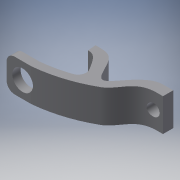
# Autodesk Inventor part: 30_Cube_Chipadapter_Fluicis_clamp
Saved by Autodesk Inventor 2019.4 (Build 234330000, 330)
## iProperties
Created: 2021-05-02
Part Number: 30_Cube_Chipadapter_Fluicis_clamp
Material: Generic
Document SubType Name: Modeling
Designer: diederichbenedict
Density: 1 g/cm^3
Appearance: Default
Author: diederichbenedict
Autodesk Inventor part; units mm, degrees
ref_plane "YZ Plane" through (0, 0, 0) normal (1, 0, 0) x (0, 1, 0)
ref_plane "XZ Plane" through (0, 0, 0) normal (0, 1, 0) x (-1, 0, 0)
ref_plane "XY Plane" through (0, 0, 0) normal (0, 0, 1) x (1, 0, 0)
sketch "Sketch1" plane through (0, 0, 0) normal (0, 1, 0) x (-1, 0, 0)
  line L0 (0, 0) -> (3.0089, 0) construction
  line L1 (3.0089, 0) -> (7.069, 5.8831) construction
  line L2 (7.069, 5.8831) -> (8.9606, 9.5326) construction
  line L3 (8.9606, 9.5326) -> (11.3861, 1.7338) construction
  line L4 (11.3861, 1.7338) -> (15.5604, 1.7338) construction
  spline S0 degree 4 poles (0, 0) (3.0089, 0) (7.069, 5.8831) (8.9606, 9.5326) (11.3861, 1.7338) (11.3861, 1.7338) (15.5604, 1.7338) knots 1 1 1 1 1 2 3 4 4 4 4 4
  line L5 (0, 0) -> (-2.509, 0)
  line L6 (-2.509, 0) -> (-2.509, 2.5)
  line L7 (-2.509, 2.5) -> (-1.0509, 2.5)
  line L8 (-1.0509, 2.5) -> (3.5176, 2.5) construction
  line L9 (3.5176, 2.5) -> (4.4785, 7.5024) construction
  line L10 (4.4785, 7.5024) -> (10.7757, 12.1884) construction
  line L11 (10.7757, 12.1884) -> (13.1491, 3.4753) construction
  line L12 (13.1491, 3.4753) -> (13.5495, 3.0077) construction
  line L13 (13.5495, 3.0077) -> (15.5604, 3.0077) construction
  spline S1 degree 4 poles (-1.0509, 2.5) (3.5176, 2.5) (4.4785, 7.5024) (10.7757, 12.1884) (13.1491, 3.4753) (13.5495, 3.0077) (15.5604, 3.0077) knots 1 1 1 1 1 2 3 4 4 4 4 4
  line L14 (15.5604, 3.0077) -> (15.5604, 1.7338)
  dimension "d0" = 2.5
  constraints: 8 end point, 5 horizontal, 2 perpendicular, 1 coincident, 6 other
  measures "d0" distance of L5.end L6.end
extrude "Extrusion1" add sketch "Sketch1" along normal blind 8
sketch "Sketch2" plane through (1.0509, 0, 2.5) normal (0, 0, 1) x (1, 0, 0)
  circle A0 centre (-0.8088, 4) radius 1.45
  line L0 (-16.6113, 8) -> (0, 8) projected
  point P0 (-1.0509, 0)
  dimension "d3" = 2.9
  dimension "d14" = 4
  constraints: 1 centre point
  measures "d3" diameter of A0
  measures "d14" distance from line of A0.centre L0
extrude "Extrusion2" cut sketch "Sketch2" along normal mid plane 7
sketch "Sketch3" plane through (0, 0, 0) normal (0, -1, 0) x (1, 0, 0)
  line L0 (2.509, 0) -> (0, 0) projected
  line L1 (2.509, 2.5) -> (2.509, 0) projected
  line L2 (1.0509, 2.5) -> (2.509, 2.5) projected
  spline S0 degree 4 poles (-15.5604, 3.0077) (-13.5495, 3.0077) (-13.1491, 3.4753) (-10.7757, 12.1884) (-4.4785, 7.5024) (-3.5176, 2.5) (1.0509, 2.5) knots 0 0 0 0 0 0.333333 0.666667 1 1 1 1 1 projected
  line L3 (-15.5604, 1.7338) -> (-15.5604, 3.0077) projected
  arc A0 (-7.1833, 8.351) -> (-19.9296, 12.3019) centre (-22.9296, -19.9129) ccw
  arc A1 (-10.767, 7.9081) -> (-19.9296, 10.3019) centre (-22.9296, -19.9129) ccw
  line L4 (-19.9296, 12.3019) -> (-19.9296, 10.3019)
  line L5 (-19.9296, 12.3019) -> (-25.9296, 12.3019)
  line L6 (-25.9296, 12.3019) -> (-25.9296, 10.3019)
  line L7 (-25.9296, 10.3019) -> (-19.9296, 10.3019)
  line L8 (-19.9296, 10.3019) -> (-19.9296, 12.3019)
  dimension "d6" = 6
  dimension "d7" = 2
  constraints: 10 end point, 5 point on circle, 2 centre point, 2 parallel, 1 concentric, 1 horizontal, 1 perpendicular, 5 other
  measures "d6" distance of L4.end L6.end
  measures "d7" distance between parallel lines of L7 L5
extrude "Extrusion3" add sketch "Sketch3" against normal up to surface (8 mm away)
sketch "Sketch4" plane through (-25.9296, 0, 12.3019) normal (0, 0, 1) x (1, 0, 0)
  arc A0 (0.3271, 6.628) -> (0.3271, 0.742) centre (3.8271, 3.685) ccw projected
  arc A1 (26.9804, 2.7965) -> (26.9804, 5.2035) centre (26.1717, 4) ccw projected
  circle A2 centre (3.8592, 4) radius 2.5
  point P0 (25.9296, 0)
  dimension "d10" = 5
  constraints: 1 centre point, 1 vertical alignment
  measures "d10" diameter of A2
extrude "Extrusion4" cut sketch "Sketch4" against normal blind 10
fillet "Fillet1" radius 2 3 edges at (-25.9296, 0, 11.3019) (-25.9296, 8, 11.3019) (-10.767, 4, 7.9081)
body "Solid1"
